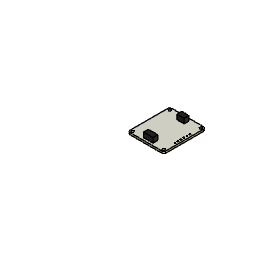
Custom PCB (Autodesk Fusion 360 design; units mm, degrees)
Autodesk Fusion 360 part; units mm, degrees
ref_plane "WorkPlane1" through (-15, -17.5, -7.5) normal (0, 0, -1) x (-1, 0, 0)
sketch "Sketch1" plane through (0, 0, -7.5) normal (0, 0, -1) x (1, 0, 0)
  arc A0 (13.4, -17.5) -> (15, -15.9) centre (13.4, -15.9) ccw
  line L0 (15, -15.9) -> (15, 15.9)
  arc A1 (15, 15.9) -> (13.4, 17.5) centre (13.4, 15.9) ccw
  line L1 (13.4, 17.5) -> (-13.4, 17.5)
  arc A2 (-13.4, 17.5) -> (-15, 15.9) centre (-13.4, 15.9) ccw
  line L2 (-15, 15.9) -> (-15, -15.9)
  arc A3 (-15, -15.9) -> (-13.4, -17.5) centre (-13.4, -15.9) ccw
  line L3 (-13.4, -17.5) -> (13.4, -17.5)
  circle A4 centre (-13, -15.5) radius 1.1
  circle A5 centre (13, 15.5) radius 1.1
  circle A6 centre (13, -15.5) radius 1.1
  circle A7 centre (-13, 15.5) radius 1.1
  line L4 (-4, 15.5) -> (-4, 11.5)
  line L5 (-4, 11.5) -> (4, 11.5)
  line L6 (4, 11.5) -> (4, 15.5)
  line L7 (4, 15.5) -> (-4, 15.5)
  line L8 (-3, -15.5) -> (3, -15.5)
  line L9 (3, -15.5) -> (3, -11.5)
  line L10 (3, -11.5) -> (-3, -11.5)
  line L11 (-3, -11.5) -> (-3, -15.5)
extrude "Extrude1" add sketch "Sketch1" along normal blind 1.6 contours A0 L0 A1 L1 A2 L2 A3 L3 | L4 L5 L6 L7 | L8 L9 L10 L11 makes body 1
extrude "Extrude1'" add sketch "Sketch1" against normal blind 4 separate body contours L4 L5 L6 L7 | L8 L9 L10 L11 makes body 2 at (1.3333, -15.5, -4.8333) makes body 3 at (-1, 12.8333, -7.5) in component "2.0mm Headers (F)"
sketch "Sketch2" plane through (0, 0, -7.5) normal (0, 0, 1) x (-1, 0, 0)
  circle A0 centre (13, -15.5) radius 1.1
  circle A1 centre (-13, 15.5) radius 1.1
  circle A2 centre (13, 15.5) radius 1.1
  circle A3 centre (-13, -15.5) radius 1.1
  line L0 (-13.4, -17.5) -> (13.4, -17.5)
  arc A4 (13.4, -17.5) -> (15, -15.9) centre (13.4, -15.9) ccw
  line L1 (15, -15.9) -> (15, 15.9)
  arc A5 (15, 15.9) -> (13.4, 17.5) centre (13.4, 15.9) ccw
  line L2 (13.4, 17.5) -> (-13.4, 17.5)
  arc A6 (-13.4, 17.5) -> (-15, 15.9) centre (-13.4, 15.9) ccw
  line L3 (-15, 15.9) -> (-15, -15.9)
  arc A7 (-15, -15.9) -> (-13.4, -17.5) centre (-13.4, -15.9) ccw
  line L4 (-13, 15.5) -> (-13, -15.5) construction
  line L5 (-13, 0) -> (-13, -1.27)
  line L6 (-13, -1.27) -> (-13, -3.81) construction
  line L7 (-13, -3.81) -> (-13, -6.35)
  line L8 (-13, 0) -> (-13, 1.27) construction
  line L9 (-13, 1.27) -> (-13, 3.81)
  line L10 (-13, 3.81) -> (-13, 6.35) construction
  circle A8 centre (-13, 3.81) radius 0.6475
  circle A9 centre (-13, 6.35) radius 0.6475
  circle A10 centre (-13, 1.27) radius 0.6475
  circle A11 centre (-13, -1.27) radius 0.6475
  circle A12 centre (-13, -3.81) radius 0.6475
  circle A13 centre (-13, -6.35) radius 0.6475
  dimension "d28_1" = 1.27
  dimension "d29_1" = 2.54
  dimension "d30_1" = 2.54
  dimension "d31_1" = 1.27
  dimension "d32_1" = 2.54
  dimension "d33_1" = 2.54
  dimension "d34" = 1.295
  dimension "d35" = 1.295
  dimension "d36" = 1.295
  dimension "d37" = 1.295
  dimension "d38" = 1.295
  dimension "d39" = 1.295
  constraint coincident A1.centre L4.start
  constraint coincident A3.centre L4.end
  constraint midpoint L4 L5.start
  constraint parallel L4 L5
  constraint parallel L4 L6
  constraint parallel L4 L7
  constraint parallel L4 L8
  constraint parallel L4 L9
  constraint parallel L4 L10
  constraint coincident L9.end L10.start
  constraint coincident L10.end A9.centre
  constraint coincident L8.end L9.start
  constraint coincident L5.end L6.start
  constraint coincident L6.end L7.start
  constraint coincident L7.end A13.centre
  measures "d28_1" distance of L5.start L5.end
  measures "d29_1" distance of L5.end L6.end
  measures "d30_1" distance of L6.end L7.end
  measures "d31_1" distance of L5.start L8.end
  measures "d32_1" distance of L8.end L9.end
  measures "d33_1" distance of L9.end L10.end
  measures "d34" diameter of A8
  measures "d35" diameter of A9
  measures "d36" diameter of A10
  measures "d37" diameter of A11
  measures "d38" diameter of A12
  measures "d39" diameter of A13
extrude "Extrude2" cut sketch "Sketch2" against normal blind 3 contours A8 | A9 | A10 | A11 | A12 | A13 bodies 1
component "2.0mm Headers (F)" placed x (1, 0, 0) y (0, 1, 0) z (0, 0, 1) at (0, 0, 0)
equation "d23_1 = 2.5 mm + 4 mm"
equation "d28_1 = ( 2.54 / 2 ) * 1 mm"
equation "d31_1 = ( 2.54 / 2 ) * 1 mm"
